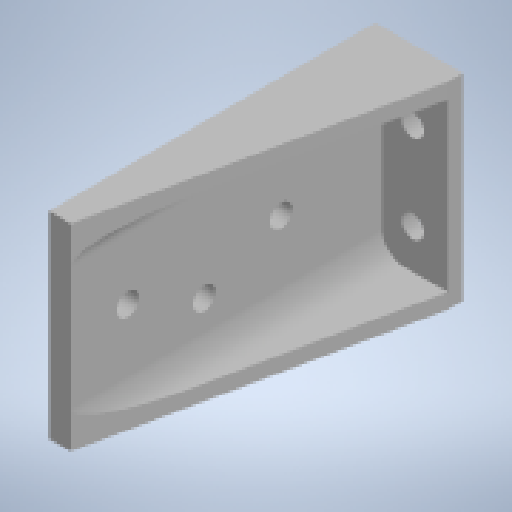
# Autodesk Inventor part: Cable_Chain_Side_Holder
Saved by Autodesk Inventor 2023 (Build 270158000, 158)
## iProperties
Created: 2023-07-02
Part Number: Cable_Chain_Side_Holder
Material: Generic
Document SubType Name: Modeling
Designer: plebbb
Density: 1 g/cm^3
Appearance: Default
Author: plebbb
Autodesk Inventor part; units mm, degrees
ref_plane "YZ Plane" through (0, 0, 0) normal (1, 0, 0) x (0, 1, 0)
ref_plane "XZ Plane" through (0, 0, 0) normal (0, 1, 0) x (-1, 0, 0)
ref_plane "XY Plane" through (0, 0, 0) normal (0, 0, 1) x (1, 0, 0)
sketch "Sketch1" plane through (0, 0, 0) normal (0, 1, 0) x (-1, 0, 0)
  line L0 (0, 0) -> (0, 71)
  line L1 (0, 71) -> (-5, 71)
  line L2 (-5, 71) -> (-20, 0)
  line L3 (-20, 0) -> (0, 0)
  dimension "d0" = 71
  dimension "d1" = 20
  dimension "d2" = 5
  constraints: 8 end point, 1 parallel, 1 perpendicular, 1 vertical
  measures "d0" distance of L0.start L0.end
  measures "d1" distance of L2.end L0.start
  measures "d2" distance of L0.end L1.end
extrude "Extrusion1" add sketch "Sketch1" along normal blind 55
sketch "Sketch2" plane through (0, 0, 0) normal (-1, 0, 0) x (0, 0, 1)
  circle A0 centre (23, 22.6) radius 2.55
  circle A1 centre (58, 22.6) radius 2.55
  circle A2 centre (40.5, 15) radius 2.55
  line L0 (23, 22.6) -> (58, 22.6) construction
  line L1 (40.5, 22.6) -> (40.5, 15) construction
  line L2 (71, 0) -> (71, 55) construction
  point P0 (0, 0)
  dimension "d5" = 5.1
  dimension "d6" = 35
  dimension "d7" = 7.6
  dimension "d8" = 15
  dimension "d9" = 30.5
  constraints: 4 end point, 3 centre point, 2 equal radius, 1 horizontal, 1 midpoint, 1 perpendicular
  measures "d5" diameter of A0
  measures "d6" distance of L0.start L0.end
  measures "d7" distance of L1.start L1.end
  measures "d8" vertical distance of L1.end point (0, 0)
  measures "d9" distance from line of L2 L1.start
extrude "Extrusion2" cut sketch "Sketch2" against normal blind 45
sketch "Sketch3" plane through (20, 0, 0) normal (0, 0, -1) x (-1, 0, 0)
  line L0 (0, 0) -> (0, 55) projected
  line L1 (0, 51.5) -> (10, 51.5)
  arc A0 (15, 46.5) -> (10, 51.5) centre (10, 46.5) ccw
  line L2 (15, 46.5) -> (15, 8.5)
  arc A1 (10, 3.5) -> (15, 8.5) centre (10, 8.5) ccw
  line L3 (10, 3.5) -> (0, 3.5)
  line L4 (15, 27.5) -> (0, 27.5) construction
  point P0 (20, 0)
  dimension "d12" = 3.5
  dimension "d13" = 3.5
  dimension "d14" = 5
  dimension "d15" = 5
  constraints: 8 end point, 4 point on circle, 3 tangent, 2 centre point, 2 horizontal, 2 midpoint, 2 point on line, 1 equal radius, 1 parallel, 1 vertical
  measures "d12" distance from line of L0.end L1
  measures "d13" distance from line of L0.start L3
  measures "d14" radius of A0
  measures "d15" distance from line of point (20, 0) L2
extrude "Extrusion3" cut sketch "Sketch3" against normal through all
sketch "Sketch5" plane through (20, 0, 0) normal (0, 0, -1) x (-1, 0, 0)
  line L0 (20, 0) -> (20, 55) projected
  line L1 (0, 55) -> (20, 55) projected
  line L2 (0, 0) -> (20, 0) projected
  line L3 (0, 51.5) -> (0, 55) projected
  line L4 (0, 55) -> (0, 0)
  constraints: 2 end point, 1 collinear
extrude "Extrusion4" add sketch "Sketch5" along normal blind 3.5
sketch "Sketch6" plane through (20, 0, 0) normal (0, 0, 1) x (1, 0, 0)
  circle A0 centre (-8, 12.5) radius 2.54
  circle A1 centre (-8, 42.5) radius 2.54
  line L0 (-8, 12.5) -> (-8, 42.5) construction
  line L1 (-20, 0) -> (-20, 55) projected
  line L2 (-20, 27.5) -> (-8, 27.5) construction
  line L3 (-15, 8.5) -> (-15, 46.5) construction
  line L4 (0, 51.5) -> (0, 3.5) construction
  line L5 (-15, 46.5) -> (-15, 8.5) projected
  line L6 (-15, 12.5) -> (-8, 12.5) construction
  line L7 (-8, 12.5) -> (0, 12.5) construction
  dimension "d20" = 5.08
  dimension "d21" = 30
  dimension "d22" = 8
  constraints: 8 end point, 2 centre point, 2 midpoint, 2 perpendicular, 2 point on line, 1 equal radius, 1 horizontal, 1 vertical
  measures "d20" diameter of A0
  measures "d21" distance of L0.start L0.end
  measures "d22" distance from line of L4 L0.start
extrude "Extrusion5" cut sketch "Sketch6" against normal through all
fillet "Fillet1" radius 3 5 edges at (6.4645, 4.9645, 0) (15, 3.5, 0) (6.4645, 50.0355, 0) (15, 51.5, 0) (5, 27.5, 0)
fillet "Fillet2" radius 3 2 edges at (12.5, 0, 35.5) (12.5, 55, 35.5)
body "Solid1"
